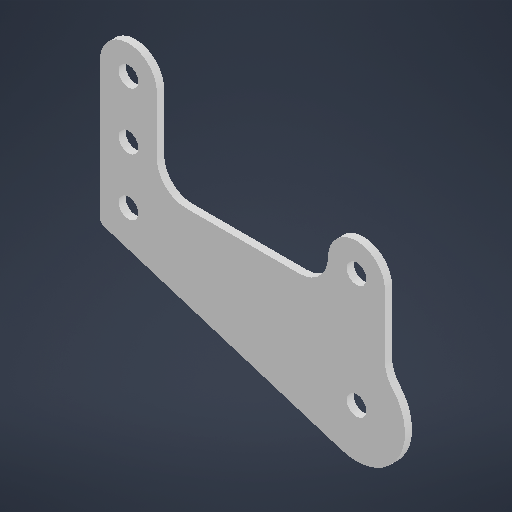
# Autodesk Inventor part: backCorners
Saved by Autodesk Inventor 2025.1 (Build 291241000, 241)
## iProperties
Created: 2025-01-10
Part Number: backCorners
Material: Generic
Document SubType Name: Modeling
Designer: Jahan
Density: 1 g/cm^3
Appearance: Default
Author: Jahan
Autodesk Inventor part; units mm, degrees
ref_plane "YZ Plane" through (0, 0, 0) normal (1, 0, 0) x (0, 1, 0)
ref_plane "XZ Plane" through (0, 0, 0) normal (0, 1, 0) x (-1, 0, 0)
ref_plane "XY Plane" through (0, 0, 0) normal (0, 0, 1) x (1, 0, 0)
sketch "Sketch1" plane through (0, 0, 0) normal (0, 0, 1) x (1, 0, 0)
  line L0 (22.6259, 3.8001) -> (22.6259, 17.6867)
  arc A0 (22.6259, 3.8001) -> (24.2707, -0.4641) centre (28.9759, 3.8001) ccw
  line L1 (3.5719, 11.3367) -> (-21.8281, 11.3367)
  arc A1 (-28.1781, 17.6867) -> (-21.8281, 11.3367) centre (-21.8281, 17.6867) ccw
  line L2 (-39.8589, -1.3663) -> (13.0314, -18.0105)
  circle A2 centre (16.2719, -7.7133) radius 2.1844
  circle A3 centre (16.2719, 17.6867) radius 2.1844
  circle A4 centre (-34.5281, 4.9867) radius 2.1844
  arc A5 (13.0314, -18.0105) -> (24.2707, -0.4641) centre (16.2719, -7.7133) ccw
  arc A6 (-40.8781, -0.3473) -> (-39.8589, -1.3663) centre (-39.3908, 0.1211) ccw
  circle A7 centre (-34.5281, 30.3867) radius 2.1844
  line L3 (-28.1781, 17.6867) -> (-28.1781, 30.3867)
  line L4 (-40.8781, 30.3867) -> (-40.8781, -0.3473)
  arc A8 (-28.1781, 30.3867) -> (-40.8781, 30.3867) centre (-34.5281, 30.3867) ccw
  arc A9 (3.5719, 11.3367) -> (9.9178, 17.6867) centre (3.5719, 17.6826) ccw
  arc A10 (22.6259, 17.6867) -> (9.9178, 17.6867) centre (16.2719, 17.6908) ccw
  circle A11 centre (-34.5281, 17.6867) radius 2.1844
  point P0 (0, 0)
  dimension "d3" = 4.3688
  constraints: 14 point on circle, 12 centre point, 10 end point, 4 tangent, 1 coincident, 1 parallel, 1 vertical
  measures "d3" diameter of A11
extrude "Extrusion2" add sketch "Sketch1" along normal blind 1.5875
body "Solid2"
